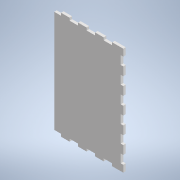
# Autodesk Inventor part: Part2
Saved by Autodesk Inventor 2022 (Build 260153000, 153)
## iProperties
Created: 2022-05-11
Part Number: Part2
Material: Generic
Document SubType Name: Modeling
Designer: Jeanette Guo
Density: 1 g/cm^3
Appearance: Default
Author: Jeanette Guo
Autodesk Inventor part; units mm, degrees
ref_plane "YZ Plane" through (0, 0, 0) normal (1, 0, 0) x (0, 1, 0)
ref_plane "XZ Plane" through (0, 0, 0) normal (0, 1, 0) x (-1, 0, 0)
ref_plane "XY Plane" through (0, 0, 0) normal (0, 0, 1) x (1, 0, 0)
sketch "Sketch1" plane through (0, 0, 0) normal (0, 0, 1) x (1, 0, 0)
  line L0 (0, 123) -> (0, 3)
  line L1 (0, 3) -> (5, 3)
  line L2 (28, 3) -> (28, 0)
  line L3 (38, 0) -> (38, 3)
  line L4 (48, 3) -> (48, 0)
  line L5 (58, 0) -> (58, 3)
  line L6 (68, 3) -> (68, 0)
  line L7 (78, 63) -> (81, 63) construction
  line L8 (0, 3) -> (5, 3)
  line L9 (78, 8) -> (78, 13)
  line L10 (78, 28) -> (78, 33)
  line L11 (78, 48) -> (78, 53)
  line L12 (78, 8) -> (78, 13)
  line L13 (81, 18) -> (81, 23)
  line L14 (78, 28) -> (78, 33)
  line L15 (78, 48) -> (78, 53)
  line L16 (81, 38) -> (81, 43)
  line L17 (81, 0) -> (81, 3) construction
  line L18 (0, 3) -> (5, 3)
  line L19 (8, 0) -> (15, 0)
  line L20 (18, 3) -> (28, 3)
  line L21 (28, 0) -> (38, 0)
  line L22 (38, 3) -> (48, 3)
  line L23 (48, 0) -> (58, 0)
  line L24 (68, 0) -> (78, 0)
  line L25 (58, 3) -> (68, 3)
  line L26 (78, 98) -> (78, 93)
  line L27 (78, 78) -> (78, 73)
  line L28 (78, 118) -> (78, 113)
  line L29 (81, 108) -> (81, 103)
  line L30 (81, 88) -> (81, 83)
  line L31 (18, 123) -> (28, 123)
  line L32 (28, 126) -> (38, 126)
  line L33 (38, 123) -> (48, 123)
  line L34 (48, 126) -> (58, 126)
  line L35 (68, 126) -> (78, 126)
  line L36 (58, 123) -> (68, 123)
  line L37 (81, 58) -> (81, 68)
  line L38 (81, 83) -> (81, 88)
  line L39 (81, 103) -> (81, 108)
  line L40 (78, 126) -> (68, 126)
  line L41 (58, 126) -> (48, 126)
  line L42 (38, 126) -> (28, 126)
  line L43 (8, 123) -> (8, 126)
  line L44 (0, 123) -> (5, 123)
  line L45 (8, 126) -> (18, 126)
  line L46 (18, 126) -> (18, 123)
  line L47 (28, 123) -> (28, 126)
  line L48 (38, 126) -> (38, 123)
  line L49 (48, 123) -> (48, 126)
  line L50 (58, 126) -> (58, 123)
  line L51 (68, 126) -> (68, 123)
  line L52 (78, 126) -> (81, 126)
  line L53 (81, 126) -> (81, 123)
  line L54 (18, 3) -> (28, 3)
  line L55 (28, 0) -> (38, 0)
  line L56 (38, 3) -> (48, 3)
  line L57 (48, 0) -> (58, 0)
  line L58 (58, 3) -> (68, 3)
  line L59 (68, 0) -> (78, 0)
  line L60 (8, 3) -> (8, 0)
  line L61 (0, 3) -> (8, 3)
  line L62 (8, 0) -> (18, 0)
  line L63 (18, 0) -> (18, 3)
  line L64 (28, 3) -> (28, 0)
  line L65 (38, 0) -> (38, 3)
  line L66 (48, 3) -> (48, 0)
  line L67 (58, 0) -> (58, 3)
  line L68 (68, 0) -> (68, 3)
  line L69 (78, 0) -> (81, 0)
  line L70 (81, 0) -> (81, 3)
  line L71 (81, 0) -> (81, 3)
  line L72 (5, 123) -> (5, 68)
  line L73 (5, 68) -> (8, 68)
  line L74 (8, 68) -> (8, 123)
  line L75 (81, 126) -> (81, 118)
  line L76 (81, 118) -> (78, 118)
  line L77 (81, 108) -> (78, 108)
  line L78 (81, 108) -> (81, 98)
  line L79 (81, 98) -> (78, 98)
  line L80 (81, 88) -> (78, 88)
  line L81 (81, 88) -> (81, 78)
  line L82 (81, 78) -> (78, 78)
  line L83 (81, 68) -> (78, 68)
  line L84 (78, 108) -> (78, 118)
  line L85 (81, 108) -> (81, 98)
  line L86 (81, 88) -> (81, 78)
  line L87 (78, 68) -> (78, 78)
  line L88 (78, 88) -> (78, 98)
  line L89 (78, 8) -> (78, 13)
  line L90 (81, 18) -> (81, 23)
  line L91 (78, 28) -> (78, 33)
  line L92 (81, 68) -> (81, 58)
  line L93 (81, 43) -> (81, 38)
  line L94 (81, 0) -> (81, 8)
  line L95 (81, 8) -> (78, 8)
  line L96 (81, 18) -> (78, 18)
  line L97 (81, 18) -> (81, 28)
  line L98 (81, 28) -> (78, 28)
  line L99 (81, 38) -> (78, 38)
  line L100 (81, 48) -> (78, 48)
  line L101 (81, 58) -> (78, 58)
  line L102 (78, 18) -> (78, 8)
  line L103 (81, 38) -> (81, 48)
  line L104 (78, 58) -> (78, 48)
  line L105 (78, 38) -> (78, 28)
  line L106 (5, 123) -> (8, 123)
  point P0 (0, 0)
  point P1 (81, 93)
  point P2 (81, 73)
  point P3 (81, 73)
  dimension "d19" = 8
  dimension "d22" = 10
  dimension "d23" = 10
  dimension "d25" = 55
  dimension "d31" = 10
  dimension "d32" = 10
  dimension "d33" = 10
  dimension "d34" = 3
  dimension "d35" = 81
  constraints: 214 end point, 33 symmetric about line, 26 perpendicular, 9 parallel, 6 collinear, 4 horizontal, 3 vertical, 1 midpoint, 1 point on line
  measures "d19" distance of L0.start L43.start
  measures "d22" distance of L43.end L45.end
  measures "d23" distance of L31.start L31.end
  measures "d25" distance of L44.end L72.end
  measures "d31" distance of L36.start L36.end
  measures "d32" distance of L34.start L34.end
  measures "d33" distance of L33.start L33.end
  measures "d34" distance of L33.end L34.start
  measures "d35" distance between parallel lines of L94 L0
extrude "Extrusion1" add sketch "Sketch1" along normal blind 3
body "Solid1"
